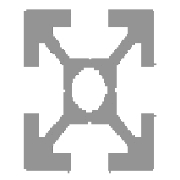
# Autodesk Inventor part: Alu Profil 20x20 - AP2020
Saved by Autodesk Inventor 2022.2 (Build 262287000, 287)
## iProperties
Created: 2022-06-05
Part Number: Alu Profil 20x20 - AP2020
Material: Generisch
Catalog Web Link: www.cadenas.de
Description: 20x20
Vendor: MISUMI
Document SubType Name: Modeling
Designer: jan
Manufacturer: MISUMI
Standards Organization: ISO
Language: de-DE
Size Designation: Alu Profil 20x20 - AP2020
Categories: <MemberInstance><Categories><Category DisplayName="Profile" InternalName="089c4875-fa83-4c05-b084-43b9cc11f5ed" Mnemonic="GRDR"><CategoryParameter DisplayName="Masse pro Längeneinheit" InternalName="0bb95a10-148f-4027-a459-38d7b056702a" Mnemonic="shpmass"/><CategoryParameter DisplayName="Querschnittsfläche" InternalName="1ff91680-64b0-4202-b9a3-7fd3f94bba3b" Mnemonic="secarea"/><CategoryParameter DisplayName="Trägheitsradius (x)" InternalName="25778675-03e9-40c1-b6a8-4a9ed693320d" Mnemonic="gyrradx"/><CategoryParameter DisplayName="Torsion-Festigkeitsmodul" InternalName="26c1ec35-5026-4c63-ad0a-751cf684a536" Mnemonic="torrigmod"/><CategoryParameter DisplayName="Abstand zum Schwerpunkt X-X" InternalName="26c9bdb8-9c79-4b4f-a92e-8e197583c9c4" Mnemonic="grcendistX"/><CategoryParameter DisplayName="Alte Varianten-ID" InternalName="340afe4f-75d7-48d3-ab7d-943f3c3da468" Mnemonic="LegacyMemberID"/><CategoryParameter DisplayName="Basislänge" InternalName="42e34263-8f20-4d0e-ad48-bf1385b87c24" Mnemonic="shplen"/><CategoryParameter DisplayName="Trägheitsmoment (y)" InternalName="4b9f58ea-bced-460e-81ea-3d29ca5a49e3" Mnemonic="inermomy"/><CategoryParameter DisplayName="Trägheitsmoment (x)" InternalName="4cd780bc-73d7-43ac-917a-579e5cbd684d" Mnemonic="inermomx"/><CategoryParameter DisplayName="Benutzerdefinierter Basispunkt" InternalName="4f1d1b73-316d-484b-a3df-9cbabb16eb77" Mnemonic="shpBasePoint"/><CategoryParameter DisplayName="Objekthöhe" InternalName="50274e7d-5ac0-4796-92cb-c59e54983c67" Mnemonic="shpheig"/><CategoryParameter DisplayName="Widerstandsmoment (y)" InternalName="59eaa5e9-d227-48dc-b6c1-6920f96e0f95" Mnemonic="secmody"/><CategoryParameter DisplayName="Schnittbezeichnung" InternalName="5a64d034-428d-49c8-ba32-7619764de20f" Mnemonic="shpdes"/><CategoryParameter DisplayName="Widerstandsmoment (x)" InternalName="72cfad18-cf51-4ed4-aaa7-c6b224f8419f" Mnemonic="secmodx"/><CategoryParameter DisplayName="Drehrissmodul" InternalName="7c55a8dc-8844-49f9-a867-cc677b30ec9a" Mnemonic="torsecmod"/><CategoryParameter DisplayName="Objektbreite" InternalName="7c717d54-a18f-4666-b4d4-573cce22c62c" Mnemonic="shpwdth"/><CategoryParameter DisplayName="Zweite Objektdicke" InternalName="9251a8e1-85fd-4e47-af99-afdb762317d9" Mnemonic="shpthick2"/><CategoryParameter DisplayName="GG Erstellt" InternalName="9c666724-f362-4ea7-ac62-f6a007de5c69" Mnemonic="shpFGAuto"/><CategoryParameter DisplayName="Abstand zum Schwerpunkt Y-Y" InternalName="bcc4fb17-7af4-436a-8f8c-d0aa3b0248c5" Mnemonic="grcendistY"/><CategoryParameter DisplayName="Trägheitsradius (y)" InternalName="bfa18ebe-1636-4dbe-8d42-b263e0b73184" Mnemonic="gyrrady"/><CategoryParameter DisplayName="Objektdicke" InternalName="d109cf76-8eb4-42fc-9800-4409734adc67" Mnemonic="shpthick"/><CategoryParameter DisplayName="Koeffizient für Schubverschiebung" InternalName="de4c90c6-aaa8-468f-a335-6737b311b5d3" Mnemonic="shdispc"/><Category DisplayName="Sonstiges" InternalName="f02205ff-2390-476f-921c-0b3185f88e84" Mnemonic="OTHSHP"><CategoryParameter DisplayName="Trägheitsmoment (y)" InternalName="044c654e-f649-48ac-84cc-650a29ae31ca" Mnemonic="inermomy"/><CategoryParameter DisplayName="Objektdicke" InternalName="12b1a788-9233-48fd-a933-2df8ff42b15f" Mnemonic="shpthick"/><CategoryParameter DisplayName="Masse pro Längeneinheit" InternalName="2fd289d6-9394-4d2d-97e6-6659d7d4551d" Mnemonic="shpmass"/><CategoryParameter DisplayName="Trägheitsradius (y)" InternalName="743e1dfe-1bba-408b-b985-cf752b207386" Mnemonic="gyrrady"/><CategoryParameter DisplayName="Widerstandsmoment (y)" InternalName="88b8bff9-a616-4028-93d5-ed4f79680d13" Mnemonic="secmody"/><CategoryParameter DisplayName="Querschnittsfläche" InternalName="c46ecdf8-b6eb-4db9-8b25-30258930c1e3" Mnemonic="secarea"/><CategoryParameter DisplayName="Widerstandsmoment (x)" InternalName="cac70804-9d39-43bb-be17-56ea1f39a6c2" Mnemonic="secmodx"/><CategoryParameter DisplayName="Trägheitsmoment (x)" InternalName="ec6737bc-264f-43ed-b0bd-f6d410c2718d" Mnemonic="inermomx"/><CategoryParameter DisplayName="Trägheitsradius (x)" InternalName="ee72c61e-565e-4fd6-b448-66e1e1abcb7e" Mnemonic="gyrradx"/></Category></Category><Category DisplayName="Datentyp" InternalName="23b78d0f-2648-40c6-8793-ca6db495c9e8" Mnemonic="DATATYPE"><CategoryParameter DisplayName="Anzeigename" InternalName="05415f3d-3907-474b-a020-eb9d644f4cf3" Mnemonic="DISPLAYNAME"/><CategoryParameter DisplayName="Norm" InternalName="0c0a119c-1e12-4c84-803f-101930972f5e" Mnemonic="STANDARD"/><CategoryParameter DisplayName="Beschreibung" InternalName="13903e3d-64b1-4950-80da-f627842ea37f" Mnemonic="DESCRIPTION"/><CategoryParameter DisplayName="Bezeichnung" InternalName="2675968c-4ce5-49e0-a4f5-552d29089031" Mnemonic="DESIGNATION"/><CategoryParameter DisplayName="Standardzeile" InternalName="2af9ec52-faaa-4026-b378-f9fa4afca842" Mnemonic="DEFAULTROW"/><CategoryParameter DisplayName="Ordnername" InternalName="3f06958e-8713-4116-9be7-ed6184ecc97b" Mnemonic="FOLDERNAME"/><CategoryParameter DisplayName="Revisionsanleitung" InternalName="45a75005-10b1-4dfc-8d6d-dfe629f0b93c" Mnemonic="REVISIONGUID"/><CategoryParameter DisplayName="Dateiname" InternalName="8b46a4cc-9585-4fed-90c3-899f57e09a73" Mnemonic="FILENAME"/><CategoryParameter DisplayName="Normungsorganisation" InternalName="8f5914e1-4693-403f-8ab5-d37768198c9d" Mnemonic="STDSORG"/><CategoryParameter DisplayName="Gruppenversion" InternalName="914462f6-6e19-4b14-ba84-155b9680b1d0" Mnemonic="FAMILYREVISION"/><CategoryParameter DisplayName="Normrevision" InternalName="91d5a463-65c2-4fde-b823-3b7fea5e8e17" Mnemonic="STANDARDREVISION"/><CategoryParameter DisplayName="Variantenrevision" InternalName="a65d44b9-392f-4f4f-857b-e4b3d54996fe" Mnemonic="MEMBERREVISION"/><CategoryParameter DisplayName="ClipFormat" InternalName="bc51e27b-3422-4e78-93ef-cec197ddf230" Mnemonic="CLIPFORMAT"/><CategoryParameter DisplayName="Hersteller" InternalName="cd6c7a72-a28a-4e50-99a9-2c7f4e13e5ad" Mnemonic="MANUFACTURER"/><CategoryParameter DisplayName="InternerName" InternalName="cf1d0246-76d9-4b4a-8305-fa0409afb5c1" Mnemonic="INTERNALNAME"/><CategoryParameter DisplayName="IstMetrisch" InternalName="e2385c5b-1ea4-4823-96a8-8de651266ec3" Mnemonic="ISMETRIC"/><Category DisplayName="Bauteil" InternalName="c0e0b642-3bcb-4cc8-9e80-f96d35c4afa4" Mnemonic="PART"><CategoryParameter DisplayName="Bauteilnummer" InternalName="016b6077-bfbe-49bd-92c9-d8d59c39c941" Mnemonic="PARTNUMBER"/><CategoryParameter DisplayName="Bestandsnummer" InternalName="4dba7c1c-e26c-444e-836c-b08b433409a8" Mnemonic="STOCKNUMBER"/><CategoryParameter DisplayName="Materialschlüssel" InternalName="5c9a8adb-dd2b-4535-b97f-0a94a95fe41f" Mnemonic="MATERIALKEY"/><CategoryParameter DisplayName="Material" InternalName="818a152a-d3c3-49ca-80ee-df7d91421b8e" Mnemonic="MATERIAL"/></Category></Category></Categories><FamilyTemplate Id="AP2020"><FamilyTemplateParameters><FamilyTemplateParameter ObjectType="kModelParameterObject" ValueType="xs:double" Id="12" ObjectReferenceKey="länge"/><FamilyTemplateParameter ObjectType="kPartComponentDefinitionObject" ValueType="xs:string" Id="23" SubObjectId="Material"/><FamilyTemplateParameter ObjectType="kPropertyObject" ValueType="xs:string" Id="26" ObjectReferenceKey="{32853F0F-3444-11d1-9E93-0060B03C1CA6}" SubObjectId="5"/><FamilyTemplateParameter ObjectType="kPropertyObject" ValueType="xs:string" Id="27" ObjectReferenceKey="{32853F0F-3444-11d1-9E93-0060B03C1CA6}" SubObjectId="52"/></FamilyTemplateParameters></FamilyTemplate><CategoryParameterMap><ParamToTemplateMap><ParamToTemplate CategoryParameter="//CategoryParameter[@InternalName='cf1d0246-76d9-4b4a-8305-fa0409afb5c1']" ConstantValue="d1642edf-44a4-4208-880b-d2c9400a76be"/><ParamToTemplate CategoryParameter="//CategoryParameter[@InternalName='45a75005-10b1-4dfc-8d6d-dfe629f0b93c']" ConstantValue="027c3718-6dee-4521-9ddb-2d6720a004f9"/><ParamToTemplate CategoryParameter="//CategoryParameter[@InternalName='3f06958e-8713-4116-9be7-ed6184ecc97b']" ConstantValue="AP"/><ParamToTemplate CategoryParameter="//CategoryParameter[@InternalName='8f5914e1-4693-403f-8ab5-d37768198c9d']" ConstantValue="ISO"/><ParamToTemplate CategoryParameter="//CategoryParameter[@InternalName='0c0a119c-1e12-4c84-803f-101930972f5e']" TemplateParameter="18"/><ParamToTemplate CategoryParameter="//CategoryParameter[@InternalName='91d5a463-65c2-4fde-b823-3b7fea5e8e17']" TemplateParameter="19"/><ParamToTemplate CategoryParameter="//CategoryParameter[@InternalName='cd6c7a72-a28a-4e50-99a9-2c7f4e13e5ad']" ConstantValue="MISUMI"/><ParamToTemplate CategoryParameter="//CategoryParameter[@InternalName='13903e3d-64b1-4950-80da-f627842ea37f']" ConstantValue="20x20"/><ParamToTemplate CategoryParameter="//CategoryParameter[@InternalName='05415f3d-3907-474b-a020-eb9d644f4cf3']" ConstantValue="AP"/><ParamToTemplate CategoryParameter="//CategoryParameter[@InternalName='914462f6-6e19-4b14-ba84-155b9680b1d0']" ConstantValue="11"/><ParamToTemplate CategoryParameter="//CategoryParameter[@InternalName='bc51e27b-3422-4e78-93ef-cec197ddf230']" ConstantValue="CF_INVENTOR.STDPARTS"/><ParamToTemplate CategoryParameter="//CategoryParameter[@InternalName='e2385c5b-1ea4-4823-96a8-8de651266ec3']" ConstantValue="true"/><ParamToTemplate CategoryParameter="//CategoryParameter[@InternalName='2af9ec52-faaa-4026-b378-f9fa4afca842']" ConstantValue="1"/><ParamToTemplate CategoryParameter="//CategoryParameter[@InternalName='9c666724-f362-4ea7-ac62-f6a007de5c69']" ConstantValue="1"/><ParamToTemplate CategoryParameter="//CategoryParameter[@InternalName='8b46a4cc-9585-4fed-90c3-899f57e09a73']" ConstantValue="Aluminium 6061-Alu Profil 20x20 - AP2020-40"/><ParamToTemplate CategoryParameter="//CategoryParameter[@InternalName='a65d44b9-392f-4f4f-857b-e4b3d54996fe']" ConstantValue="a80eac76-ed7a-4b6c-a430-4b848d6684e2"/><ParamToTemplate CategoryParameter="//CategoryParameter[@InternalName='a65d44b9-392f-4f4f-857b-e4b3d54996fe']" ConstantValue="a80eac76-ed7a-4b6c-a430-4b848d6684e2"/><ParamToTemplate CategoryParameter="//CategoryParameter[@InternalName='2675968c-4ce5-49e0-a4f5-552d29089031']" TemplateParameter="27"/><ParamToTemplate CategoryParameter="//CategoryParameter[@InternalName='818a152a-d3c3-49ca-80ee-df7d91421b8e']" TemplateParameter="23"/><ParamToTemplate CategoryParameter="//CategoryParameter[@InternalName='016b6077-bfbe-49bd-92c9-d8d59c39c941']" TemplateParameter="26"/><ParamToTemplate CategoryParameter="//CategoryParameter[@InternalName='42e34263-8f20-4d0e-ad48-bf1385b87c24']" TemplateParameter="12"/></ParamToTemplateMap></CategoryParameterMap></MemberInstance>
Mass: 10.3404 g
Surface Area: 109.756 cm^2
Volume: 10.3404 cm^3
Density: 1 g/cm^3
Appearance: Vorgabe
_CCFamilyDisplayName: AP - 20x20
_FrameMemberDoc: Frame Member File
_Version: 15.0.0
_GetPNFromCC: 1
Company: MISUMI
IsCustomPart: 1
PSOL_IDENT_0: {$CADENAS_DATA\23d-libs\misumi\metric\38_al_extrusions_blackets\5\khfs5_2020.prj},309 {VTYP=3D},{NB=
PSOL_IDENT_1: KHFS5-2020-4000},{LINA=KHFS5-2020-4000},{NN=KHFS5-2020-4000, KHFSB5-2020-4000, KHFSF5-2020-4000, KHF
PSOL_IDENT_2: SFB5-2020-4000, KHFST5-2020-4000, KHFSTB5-2020-4000, KHFSH5-2020-4000, KHFSC5-2020-4000},{DATE=17.07
PSOL_IDENT_3: .2015 10:47:11},{GEOMDATE=07.04.2011 07:46:00},{VERSION=},{LINEID=10},{LINESUBID=-1},{WBVAR=}  {NB=K
PSOL_IDENT_4: HFS5-2020-4000},{LINA=KHFS5-2020-4000},{KT=1},{PN=KHFS5-2020-4000},{TPS=KHFS5-2020},{TP=KHFS5},{FRM=
PSOL_IDENT_5: 2020},{MAT=A6N01SS-T5 Aluminum Alloy or 6005A-T5 Aluminum Alloy},{ST=Clear Anodize},{FEAT=Four-Side
PSOL_IDENT_6: Slots},{L=4000},{LTOL=+/- 0.5},{MASS=0},{SA=183},{GMILX=0.742x10^4},{GMILY=0.742x10^4},{CLF=HFS5-202
PSOL_IDENT_7: 0},{WIDTH=20.000},{HEIGHT=20.000},{VER=1},{DIM=1},{DRILLDIA=4.200}
NN: KHFS5-2020-4000, KHFSB5-2020-4000, KHFSF5-2020-4000, KHFSFB5-2020-4000, KHFST5-2020-4000, KHFSTB5-2020-4000, KHFSH5-2020-4000, KHFSC5-2020-4000
NT: HFS5 Series Aluminum Extrusions 20,25,40mm Square -1 Slot-
NB: KHFS5-2020-4000
NBSYN: $PN.
LINA: KHFS5-2020-4000
PN: KHFS5-2020-4000
TPS: KHFS5-2020
MAT: A6N01SS-T5 Aluminum Alloy or 6005A-T5 Aluminum Alloy
ST: Clear Anodize
L: 4000
LTOL: +/- 0.5
SA: 183
GMILX: 0.742x10^4
GMILY: 0.742x10^4
CLF: HFS5-2020
SUPPLIER: MISUMI
ARTICLENO: KHFS5-2020-4000
BOMINFO: KHFS5-2020-4000
CREATOR: CADENAS GmbH
G_L: 60,000 mm
G_W: 20,000 mm
G_H: 20,000 mm
Title: KHFS5-2020-4000
Author: jan
Comments: HFS5 Series Aluminum Extrusions 20,25,40mm Square -1 Slot-
Autodesk Inventor part; units mm, degrees
ref_plane "Startebene" through (0, 0, 0) normal (0, 0, 1) x (1, 0, 0)
ref_plane "Endebene" through (0, 0, 320) normal (0, 0, 1) x (1, 0, 0)
ref_plane "Startebene1" through (0, 0, 0) normal (0, 0, 1) x (1, 0, 0)
ref_plane "Endebene1" through (0, 0, 40) normal (0, 0, 1) x (1, 0, 0)
ref_plane "Startebene2" through (0, 0, 0) normal (0, 0, 1) x (1, 0, 0)
ref_plane "Endebene2" through (0, 0, 40) normal (0, 0, 1) x (1, 0, 0)
ref_plane "Startebene3" through (0, 0, 0) normal (0, 0, 1) x (1, 0, 0)
ref_plane "Endebene3" through (0, 0, 60) normal (0, 0, 1) x (1, 0, 0)
sketch "Skizze" plane through (0, 0, 0) normal (0, 0, 1) x (1, 0, 0)
  line L0 (-10, 9) -> (-10, 3.3)
  arc A0 (-10, 3.3) -> (-9.7, 3) centre (-9.7, 3.3) ccw
  line L1 (-9.7, 3) -> (-8, 3)
  line L2 (-8, 3) -> (-8, 6)
  line L3 (-8, 6) -> (-7.0607, 6)
  line L4 (-7.0607, 6) -> (-4, 2.9393)
  line L5 (-4, 2.9393) -> (-4, 0.3)
  line L6 (-4, 0.3) -> (-3.7, 0)
  line L7 (-3.7, 0) -> (-4, -0.3)
  line L8 (-4, -0.3) -> (-4, -2.9393)
  line L9 (-4, -2.9393) -> (-7.0607, -6)
  line L10 (-7.0607, -6) -> (-8, -6)
  line L11 (-8, -6) -> (-8, -3)
  line L12 (-8, -3) -> (-9.7, -3)
  arc A1 (-9.7, -3) -> (-10, -3.3) centre (-9.7, -3.3) ccw
  line L13 (-10, -3.3) -> (-10, -9)
  arc A2 (-10, -9) -> (-9, -10) centre (-9, -9) ccw
  line L14 (-9, -10) -> (-3.3, -10)
  arc A3 (-3.3, -10) -> (-3, -9.7) centre (-3.3, -9.7) ccw
  line L15 (-3, -9.7) -> (-3, -8)
  line L16 (-3, -8) -> (-6, -8)
  line L17 (-6, -8) -> (-6, -7.0607)
  line L18 (-6, -7.0607) -> (-2.9393, -4)
  line L19 (-2.9393, -4) -> (-0.3, -4)
  line L20 (-0.3, -4) -> (0, -3.7)
  line L21 (0, -3.7) -> (0.3, -4)
  line L22 (0.3, -4) -> (2.9393, -4)
  line L23 (2.9393, -4) -> (6, -7.0607)
  line L24 (6, -7.0607) -> (6, -8)
  line L25 (6, -8) -> (3, -8)
  line L26 (3, -8) -> (3, -9.7)
  arc A4 (3, -9.7) -> (3.3, -10) centre (3.3, -9.7) ccw
  line L27 (3.3, -10) -> (9, -10)
  arc A5 (9, -10) -> (10, -9) centre (9, -9) ccw
  line L28 (10, -9) -> (10, -3.3)
  arc A6 (10, -3.3) -> (9.7, -3) centre (9.7, -3.3) ccw
  line L29 (9.7, -3) -> (8, -3)
  line L30 (8, -3) -> (8, -6)
  line L31 (8, -6) -> (7.0607, -6)
  line L32 (7.0607, -6) -> (4, -2.9393)
  line L33 (4, -2.9393) -> (4, -0.3)
  line L34 (4, -0.3) -> (3.7, 0)
  line L35 (3.7, 0) -> (4, 0.3)
  line L36 (4, 0.3) -> (4, 2.9393)
  line L37 (4, 2.9393) -> (7.0607, 6)
  line L38 (7.0607, 6) -> (8, 6)
  line L39 (8, 6) -> (8, 3)
  line L40 (8, 3) -> (9.7, 3)
  arc A7 (9.7, 3) -> (10, 3.3) centre (9.7, 3.3) ccw
  line L41 (10, 3.3) -> (10, 9)
  arc A8 (10, 9) -> (9, 10) centre (9, 9) ccw
  line L42 (9, 10) -> (3.3, 10)
  arc A9 (3.3, 10) -> (3, 9.7) centre (3.3, 9.7) ccw
  line L43 (3, 9.7) -> (3, 8)
  line L44 (3, 8) -> (6, 8)
  line L45 (6, 8) -> (6, 7.0607)
  line L46 (6, 7.0607) -> (2.9393, 4)
  line L47 (2.9393, 4) -> (0.3, 4)
  line L48 (0.3, 4) -> (0, 3.7)
  line L49 (0, 3.7) -> (-0.3, 4)
  line L50 (-0.3, 4) -> (-2.9393, 4)
  line L51 (-2.9393, 4) -> (-6, 7.0607)
  line L52 (-6, 7.0607) -> (-6, 8)
  line L53 (-6, 8) -> (-3, 8)
  line L54 (-3, 8) -> (-3, 9.7)
  arc A10 (-3, 9.7) -> (-3.3, 10) centre (-3.3, 9.7) ccw
  line L55 (-3.3, 10) -> (-9, 10)
  arc A11 (-9, 10) -> (-10, 9) centre (-9, 9) ccw
  circle A12 centre (0, 0) radius 2.75
  dimension "d2" = 5.5
  dimension "d3" = 10
  dimension "d4" = 10
  dimension "d5" = 5.7
  dimension "d6" = 5.7
  dimension "d7" = 1.7
  dimension "d8" = 3
  dimension "d9" = 0.3
  dimension "d10" = 90
  dimension "d11" = 45
  dimension "d12" = 45
  dimension "d13" = 45
  dimension "d14" = 90
  dimension "d15" = 90
  dimension "d16" = 45
  dimension "d17" = 45
  dimension "d18" = 45
  dimension "d19" = 45
  dimension "d20" = 90
  dimension "d21" = 90
  dimension "d22" = 45
  dimension "d23" = 45
  dimension "d24" = 90
  dimension "d25" = 90
  dimension "d26" = 90
  dimension "d27" = 90
  dimension "d28" = 90
  dimension "d29" = 90
  dimension "d30" = 90
  dimension "d31" = 90
  dimension "d32" = 90
  dimension "d33" = 90
  dimension "d34" = 90
  dimension "d35" = 90
  dimension "d36" = 90
  dimension "d37" = 90
  dimension "d38" = 90
  dimension "d39" = 4
  dimension "d40" = 6
  dimension "d41" = 13
  dimension "d42" = 14
  dimension "d43" = 16
  dimension "d44" = 18
  dimension "d45" = 3
  dimension "d46" = 9
  dimension "d47" = 7
  dimension "d48" = 1
  dimension "d49" = 7
  dimension "d50" = 1.5
  dimension "d51" = 1.8663
  dimension "d52" = 3.3663
  dimension "d53" = 1.5
  dimension "d54" = 1.8663
  dimension "d55" = 3.3663
  dimension "d56" = 4
  dimension "d57" = 10.8187
  dimension "d58" = 1.9092
  dimension "d59" = 5
  dimension "d60" = 13
  dimension "d61" = 13
  dimension "d62" = 16.0513
  dimension "d63" = 3.3234
  dimension "d64" = 14
  dimension "d65" = 12.685
  constraints: 112 end point, 32 tangent, 24 point on circle, 23 parallel, 20 equal length, 13 centre point, 4 equal radius, 1 coincident, 1 horizontal, 1 perpendicular, 1 vertical
  measures "d2" diameter of A12
  measures "d3" distance from line of point (0, 0) L42
  measures "d4" distance from line of L14 point (0, 0)
  measures "d5" distance of L13.start L13.end
  measures "d6" distance of L0.start L0.end
  measures "d7" distance of L1.start L1.end
  measures "d8" vertical distance of L1.end A12.centre
  measures "d9" radius of A7
  measures "d10" angle of L41 L40
  measures "d11" angle of L41 L37
  measures "d12" angle of L49 L41
  measures "d13" angle of L20 L41
  measures "d14" angle of L50 L41
  measures "d15" angle of L19 L41
  measures "d16" angle of L6 L41
  measures "d17" angle of L7 L41
  measures "d18" angle of L41 L51
  measures "d19" angle of L41 L18
  measures "d20" angle of L53 L41
  measures "d21" angle of L16 L41
  measures "d22" angle of L41 L4
  measures "d23" angle of L41 L9
  measures "d24" angle of L41 L55
  measures "d25" angle of L41 L14
  measures "d26" angle of L3 L41
  measures "d27" angle of L10 L41
  measures "d28" angle of L1 L41
  measures "d29" angle of L41 L12
  measures "d30" angle of L39 L40
  measures "d31" angle of L45 L40
  measures "d32" angle of L36 L40
  measures "d33" angle of L43 L40
  measures "d34" angle of L54 L40
  measures "d35" angle of L5 L40
  measures "d36" angle of L52 L40
  measures "d37" angle of L2 L40
  measures "d38" angle of L0 L40
  measures "d39" distance between parallel lines of L24 L28
  measures "d40" distance between parallel lines of L33 L28
  measures "d41" distance between parallel lines of L15 L28
  measures "d42" distance between parallel lines of L8 L28
  measures "d43" distance between parallel lines of L17 L28
  measures "d44" distance between parallel lines of L11 L28
  measures "d45" distance between parallel lines of L38 L40
  measures "d46" distance between parallel lines of L31 L40
  measures "d47" distance between parallel lines of L42 L40
  measures "d48" distance between parallel lines of L47 L40
  measures "d49" distance between parallel lines of L22 L40
  measures "d50" distance between parallel lines of L46 L37
  measures "d51" distance between parallel lines of L35 L37
  measures "d52" distance between parallel lines of L48 L37
  measures "d53" distance between parallel lines of L23 L32
  measures "d54" distance between parallel lines of L34 L32
  measures "d55" distance between parallel lines of L21 L32
  measures "d56" distance from line of L41.end L45
  measures "d57" distance from line of L41.end L49
  measures "d58" distance from line of L41.end L20
  measures "d59" distance from line of L41.end L50
  measures "d60" distance from line of L41.end L19
  measures "d61" distance from line of L41.end L54
  measures "d62" distance from line of L41.end L6
  measures "d63" distance from line of L41.end L7
  measures "d64" distance from line of L41.end L5
  measures "d65" distance from line of L41.end L51
extrude "Körper" add sketch "Skizze" along normal up to surface (60 mm away) from surface at 0
sketch "Skizze21" plane through (0, 0, 0) normal (0, 0, 1) x (1, 0, 0)
  line L0 (0, 0) -> (10, 0)
ref_plane "Arbeitsebene18" through (0, 0, 0) normal (0, -1, 0) x (1, 0, 0)
sketch "Skizze22" plane through (0, 0, 0) normal (0, -1, 0) x (1, 0, 0)
  line L0 (-2, 0) -> (12, 0)
  line L1 (-2, 60) -> (12, 60)
  dimension "d80" = 60
  measures "d80" distance between parallel lines of L0 L1
equation "\"G_OFFSET_START\" = 0"
equation "\"G_OFFSET_END\" = 0"
equation "\"G_L\" = d80"
equation "\"G_OFFSET_START1\" = 0"
equation "\"G_OFFSET_END1\" = 0"
equation "\"G_OFFSET_START2\" = 0"
equation "\"G_OFFSET_END2\" = 0"
equation "\"G_OFFSET_START3\" = 0"
equation "\"G_OFFSET_END3\" = 0"
body "Solid1"
